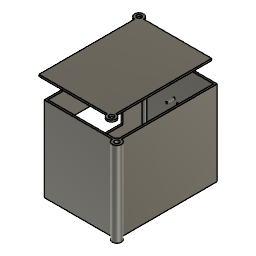
trabajo TEO grupo 5 (Autodesk Fusion 360 design; units mm, degrees)
part number: 2026-06-23-14-01-29-203
Autodesk Fusion 360 part; units mm, degrees
sketch "Boceto1" plane through (0, 0, 0) normal (0, 0, 1) x (1, 0, 0)
  line L0 (0, 0) -> (-75, 0)
  line L1 (-75, 0) -> (-75, -105)
  line L2 (-75, -105) -> (0, -105)
  line L3 (0, -105) -> (0, 0)
  dimension "d1" = 75
  dimension "d2" = 105
  constraint horizontal L0
  constraint vertical L1
  constraint horizontal L2
  constraint vertical L3
  constraint coincident L0.start L3.end
  measures "d1" distance of L0.start L0.end
  measures "d2" distance of L0.start L2.end
extrude "Extruir1" add sketch "Boceto1" along normal blind 90 makes body 1
sketch "Boceto2" plane through (-75, 0, 0) normal (-1, 0, 0) x (0, -1, 0)
  line L0 (0, 0) -> (105, 0)
  line L1 (105, 0) -> (105, 90)
  line L2 (105, 90) -> (0, 90)
  line L3 (0, 90) -> (0, 0)
shell "Vaciado1" thickness 2 outward yes removed faces 1 at (-50, -35, 90) on bodies 1
sketch "Boceto3" plane through (-77, 0, 0) normal (-1, 0, 0) x (0, -1, 0)
  line L0 (-2, -2) -> (107, -2)
  line L1 (107, -2) -> (107, 90)
  line L2 (107, 90) -> (-2, 90)
  line L3 (-2, 90) -> (-2, -2)
sketch "Boceto4" plane through (-75, 0, 0) normal (-1, 0, 0) x (0, -1, 0)
sketch "Boceto5" plane through (0, 0, 0) normal (0, -1, 0) x (1, 0, 0)
  line L0 (-75, 0) -> (0, 0)
  line L1 (0, 0) -> (0, 90)
  line L2 (0, 90) -> (-75, 90)
  line L3 (-75, 90) -> (-75, 0)
  line L4 (-75, 90) -> (0, 90)
  line L5 (-37.5, 90) -> (-37.5, 55)
  line L6 (-37.5, 55) -> (-35, 55)
  line L7 (-37.5, 55) -> (-40, 55)
  line L8 (-40, 55) -> (-40, 40.25)
  line L9 (-40, 55) -> (-35, 55)
  line L10 (-35, 55) -> (-35, 40.25)
  line L11 (-35, 40.25) -> (-40, 40.25)
  line L12 (-40, 40.25) -> (-40, 55)
  dimension "d6" = 35
  dimension "d7" = 2.5
  dimension "d8" = 2.5
  dimension "d9" = 14.75
  constraint coincident L2.end L3.start
  constraint coincident L1.end L2.start
  constraint midpoint L4 L5.start
  constraint perpendicular L2 L5
  constraint perpendicular L5 L6
  constraint perpendicular L5 L7
  constraint perpendicular L7 L8
  constraint horizontal L9
  constraint vertical L10
  constraint horizontal L11
  constraint vertical L12
  measures "d6" distance of L5.start L5.end
  measures "d7" distance of L5.end L6.end
  measures "d8" distance of L5.end L7.end
  measures "d9" distance of L7.end L8.end
extrude "Extruir2" cut sketch "Boceto5" along normal blind 0 and the other way blind 4 contours L6 L7 L8 L9 L10 L11 L12 bodies 1
sketch "Boceto6" plane through (0, 2, 0) normal (0, 1, 0) x (-1, 0, 0)
  line L0 (35, 40.25) -> (35, 55)
  line L1 (35, 55) -> (40, 55)
  line L2 (40, 55) -> (40, 40.25)
  line L3 (40, 40.25) -> (35, 40.25)
  line L4 (-2, -2) -> (77, -2)
  line L5 (77, -2) -> (77, 90)
  line L6 (77, 90) -> (-2, 90)
  line L7 (-2, 90) -> (-2, -2)
  line L8 (37.5, 55) -> (41.7, 55)
  line L9 (37.5, 55) -> (33.3, 55)
  circle A0 centre (32.21, 55) radius 1.09
  circle A1 centre (42.79, 55) radius 1.09
  line L10 (35, 55) -> (35, 51)
  dimension "d14" = 4.2
  dimension "d15" = 4.2
  dimension "d16" = 2.18
  dimension "d17" = 2.18
  dimension "d18" = 4
  constraint midpoint L1 L8.start
  constraint parallel L1 L8
  constraint parallel L1 L9
  constraint coincident L9.end A0
  constraint coincident L8.end A1
  constraint coincident L0.end L1.start
  constraint perpendicular L9 L10
  measures "d14" distance of L8.start L8.end
  measures "d15" distance of L8.start L9.end
  measures "d16" diameter of A0
  measures "d17" diameter of A1
  measures "d18" distance of L0.end L10.end
extrude "Extruir3" add 1 faces at (-36.6667, 0.6667, 55) along direction (0, 0, -1) blind 2.5 on bodies 1 bodies 1
extrude "Extruir4" cut sketch "Boceto6" along normal blind 0 and the other way blind 3 contours A0 bodies 1
extrude "Extruir5" cut sketch "Boceto6" against normal blind 3.5 contours A1 bodies 1
sketch "Boceto7" plane through (0, 0, -2) normal (0, 0, -1) x (1, 0, 0)
  line L0 (2, -2) -> (2, 107)
  line L1 (2, 107) -> (-77, 107)
  line L2 (-77, 107) -> (-77, -2)
  line L3 (-77, -2) -> (2, -2)
sketch "Boceto8" plane through (-75, 0, 0) normal (-1, 0, 0) x (0, -1, 0)
  line L0 (105, 90) -> (0, 90)
  line L1 (52.5, 90) -> (52.5, 60.8734)
  line L2 (52.5, 60.8734) -> (23.5, 60.8734)
  line L3 (52.5, 60.8734) -> (81.5, 60.8734)
  line L4 (23.5, 60.8734) -> (23.5, 25.8734)
  line L5 (23.5, 60.8734) -> (81.5, 60.8734)
  line L6 (81.5, 60.8734) -> (81.5, 25.8734)
  line L7 (81.5, 25.8734) -> (23.5, 25.8734)
  line L8 (23.5, 25.8734) -> (23.5, 60.8734)
  dimension "d27" = 29
  dimension "d28" = 29
  dimension "d29" = 35
  constraint midpoint L0 L1.start
  constraint perpendicular L0 L1
  constraint perpendicular L1 L2
  constraint perpendicular L1 L3
  constraint perpendicular L2 L4
  constraint horizontal L5
  constraint vertical L6
  constraint horizontal L7
  constraint vertical L8
  measures "d27" distance of L1.end L2.end
  measures "d28" distance of L1.end L3.end
  measures "d29" distance of L2.end L4.end
extrude "Extruir6" cut sketch "Boceto8" along normal blind 19 bodies 1
sketch "Boceto9" plane through (0, 0, 0) normal (0, 0, 1) x (-1, 0, 0)
  line L0 (0, 105) -> (0, 0)
  line L1 (0, 0) -> (75, 0)
  line L2 (75, 0) -> (75, 105)
  line L3 (75, 105) -> (0, 105)
  line L4 (37.5, 105) -> (37.5, 0)
  circle A0 centre (37.5, 52.5) radius 9.725
  line L5 (-2, -2, -2) -> (-2, 107, -2)
  line L6 (-2, 107, -2) -> (77, 107, -2)
  line L7 (77, 107, -2) -> (77, -2, -2)
  line L8 (77, -2, -2) -> (-2, -2, -2)
  dimension "d32" = 19.45
  constraint midpoint L3 L4.start
  constraint midpoint L1 L4.end
  constraint midpoint L4 A0.centre
  measures "d32" diameter of A0
extrude "Extruir7" cut sketch "Boceto9" along normal blind -25 and the other way blind 0 contours L4 A0 | L4 A0 bodies 1
sketch "Boceto10" plane through (0, 0, 0) normal (0, 0, 1) x (-1, 0, 0)
  circle A0 centre (37.5, 52.5) radius 9.725
  line L0 (0, 105) -> (0, 0)
  line L1 (0, 0) -> (75, 0)
  line L2 (75, 0) -> (75, 105)
  line L3 (75, 105) -> (0, 105)
  line L4 (30.6188, 59.3721) -> (44.3812, 59.3721)
  line L5 (28.7722, 56.7896) -> (46.2278, 56.7896)
  line L6 (27.775, 52.5) -> (47.225, 52.5)
  line L7 (28.7699, 48.215) -> (46.2301, 48.215)
  line L8 (31.7733, 44.64) -> (43.2267, 44.64)
  constraint coincident A0 L4.start
  constraint coincident A0 L4.end
  constraint horizontal L4
  constraint coincident A0 L5.start
  constraint coincident A0 L5.end
  constraint parallel L4 L5
  constraint coincident A0 L6.start
  constraint coincident A0 L6.end
  constraint parallel L5 L6
  constraint coincident A0 L7.start
  constraint coincident A0 L7.end
  constraint parallel L5 L7
  constraint coincident A0 L8.start
  constraint coincident A0 L8.end
  constraint parallel L7 L8
extrude "Extruir8" add sketch "Boceto10" against normal blind 2 contours A0 L6 L7 | A0 L4 L5 | A0 L8 bodies 1
sketch "Boceto11" plane through (0, 0, 0) normal (0, 0, 1) x (-1, 0, 0)
  arc A0 (43.2267, 44.64) -> (46.2301, 48.215) centre (37.5, 52.5) ccw
  line L0 (43.2267, 44.64) -> (31.7733, 44.64)
  arc A1 (28.7699, 48.215) -> (31.7733, 44.64) centre (37.5, 52.5) ccw
  line L1 (28.7699, 48.215) -> (46.2301, 48.215)
  line L2 (47.225, 52.5) -> (27.775, 52.5)
  arc A2 (28.7722, 56.7896) -> (27.775, 52.5) centre (37.5, 52.5) ccw
  line L3 (28.7722, 56.7896) -> (46.2278, 56.7896)
  arc A3 (47.225, 52.5) -> (46.2278, 56.7896) centre (37.5, 52.5) ccw
  line L4 (44.3812, 59.3721) -> (30.6188, 59.3721)
  arc A4 (44.3812, 59.3721) -> (30.6188, 59.3721) centre (37.5, 52.5) ccw
  line L5 (0, 105) -> (0, 0)
  line L6 (0, 0) -> (75, 0)
  line L7 (75, 0) -> (75, 105)
  line L8 (75, 105) -> (0, 105)
  line L9 (31.0217, 64.79) -> (43.5417, 64.79)
  circle A5 centre (44.9317, 64.79) radius 1.39
  circle A6 centre (29.6317, 64.79) radius 1.39
  line L10 (29.6819, 63.4009) -> (29.6819, 38.6409)
  line L11 (44.9317, 63.4) -> (44.9317, 38.64)
  circle A7 centre (29.6819, 37.2509) radius 1.39
  circle A8 centre (44.9317, 37.25) radius 1.39
  dimension "d39" = 12.52
  dimension "d40" = 2.78
  dimension "d41" = 2.78
  dimension "d42" = 24.76
  dimension "d43" = 24.76
  dimension "d44" = 2.78
  dimension "d45" = 2.78
  constraint horizontal L9
  constraint coincident L9.end A5
  constraint coincident L9.start A6
  constraint coincident A6 L10.start
  constraint perpendicular L1 L10
  constraint coincident A5 L11.start
  constraint vertical L11
  constraint coincident L10.end A7
  constraint coincident L11.end A8
  measures "d39" distance of L9.start L9.end
  measures "d40" diameter of A5
  measures "d41" diameter of A6
  measures "d42" distance of L10.start L10.end
  measures "d43" distance of L11.start L11.end
  measures "d44" diameter of A7
  measures "d45" diameter of A8
extrude "Extruir9" cut sketch "Boceto11" along normal blind -4 and the other way blind 0 contours A5 | A6 | A7 | A8 bodies 1
sketch "Boceto12" plane through (-75, 0, 0) normal (-1, 0, 0) x (0, -1, 0)
  line L0 (23.5, 25.8734) -> (81.5, 25.8734)
  line L1 (52.5, 25.8734) -> (52.5, 23.9434)
  circle A0 centre (52.5, 21.7434) radius 2.2
  dimension "d50" = 1.93
  dimension "d51" = 4.4
  constraint midpoint L0 L1.start
  constraint perpendicular L0 L1
  constraint coincident L1.end A0
  measures "d50" distance of L1.start L1.end
  measures "d51" diameter of A0
extrude "Extruir10" add sketch "Boceto12" against normal blind 19 bodies 1
sketch "Boceto13" plane through (0, 0, 0) normal (0, 0, 1) x (-1, 0, 0)
  line L0 (0, 105) -> (0, 0)
  line L1 (0, 0) -> (75, 0)
  line L2 (75, 0) -> (75, 105)
  line L3 (75, 105) -> (0, 105)
  line L4 (44.3812, 59.3721) -> (30.6188, 59.3721)
  arc A0 (44.3812, 59.3721) -> (30.6188, 59.3721) centre (37.5, 52.5) ccw
  line L5 (47.225, 52.5) -> (27.775, 52.5)
  arc A1 (28.7722, 56.7896) -> (27.775, 52.5) centre (37.5, 52.5) ccw
  line L6 (28.7722, 56.7896) -> (46.2278, 56.7896)
  arc A2 (47.225, 52.5) -> (46.2278, 56.7896) centre (37.5, 52.5) ccw
  arc A3 (43.2267, 44.64) -> (46.2301, 48.215) centre (37.5, 52.5) ccw
  line L7 (43.2267, 44.64) -> (31.7733, 44.64)
  arc A4 (28.7699, 48.215) -> (31.7733, 44.64) centre (37.5, 52.5) ccw
  line L8 (28.7699, 48.215) -> (46.2301, 48.215)
  circle A5 centre (29.6819, 37.2509) radius 1.39
  circle A6 centre (44.9317, 64.79) radius 1.39
  circle A7 centre (44.9317, 37.25) radius 1.39
  circle A8 centre (29.6317, 64.79) radius 1.39
  circle A9 centre (29.6819, 37.2509) radius 1.39
  circle A10 centre (44.9317, 37.25) radius 1.39
  circle A11 centre (44.9317, 64.79) radius 1.39
  circle A12 centre (29.6317, 64.79) radius 1.39
  constraint concentric A5 A9
  constraint concentric A7 A10
  constraint concentric A6 A11
  constraint concentric A8 A12
extrude "Extruir11" add sketch "Boceto13" along normal blind 23 separate body contours A5 A9 | A6 A11 | A7 A10 | A8 A12 makes body 2 at (-46.3199, -37.1808, 15.3333) makes body 3 at (-31.0702, -37.1817, 15.3333) makes body 4 at (-28.2434, -64.8593, 15.3333) makes body 5 at (-46.1524, -65.4548, 7.6667)
extrude "Extruir12" add sketch "Boceto6" along normal blind 0 and the other way blind 10 contours A0 | A1 bodies 1
sketch "Boceto14" plane through (0, 0, -2) normal (0, 0, -1) x (1, 0, 0)
  circle A0 centre (1.9998, 106.9999) radius 5
  circle A1 centre (-76.9997, -1.9997) radius 5
  dimension "d60" = 10
  dimension "d61" = 10
  measures "d60" diameter of A0
  measures "d61" diameter of A1
extrude "Extruir13" add sketch "Boceto14" along normal blind 0 and the other way blind 92 bodies 1
sketch "Boceto15" plane through (0, 0, 90) normal (0, 0, 1) x (-1, 0, 0)
  line L0 (2.5828, 105) -> (75, 105)
  line L1 (75, 105) -> (75, 2.583)
  arc A0 (75, 2.583) -> (72.417, 0) centre (76.9997, -1.9997) ccw
  line L2 (72.417, 0) -> (0, 0)
  line L3 (0, 0) -> (0, 102.4172)
  arc A1 (0, 102.4172) -> (2.5828, 105) centre (-1.9998, 106.9999) ccw
  arc A2 (3.0002, 107) -> (-2, 101.9999) centre (-1.9998, 106.9999) ccw
  line L4 (-2, 101.9999) -> (-2, -2)
  line L5 (-2, -2) -> (71.9997, -2)
  arc A3 (71.9997, -2) -> (77, 3.0003) centre (76.9997, -1.9997) ccw
  line L6 (77, 3.0003) -> (77, 107)
  line L7 (77, 107) -> (3.0002, 107)
  circle A4 centre (76.9997, -1.9997) radius 2.5
  circle A5 centre (-1.9998, 106.9999) radius 2.5
  dimension "d66" = 5
  dimension "d67" = 5
  constraint concentric A0 A4
  constraint concentric A1 A5
  measures "d66" diameter of A4
  measures "d67" diameter of A5
extrude "Extruir14" cut sketch "Boceto15" against normal blind 4 contours A4 | A5 bodies 1
sketch "Boceto16" plane through (0, 0, 90) normal (0, 0, 1) x (-1, 0, 0)
  circle A0 centre (-1.9998, 106.9999) radius 2.5
  circle A1 centre (76.9997, -1.9997) radius 2.5
  line L0 (2.5828, 105) -> (75, 105)
  line L1 (75, 105) -> (75, 2.583)
  arc A2 (75, 2.583) -> (72.417, 0) centre (76.9997, -1.9997) ccw
  line L2 (72.417, 0) -> (0, 0)
  line L3 (0, 0) -> (0, 102.4172)
  arc A3 (0, 102.4172) -> (2.5828, 105) centre (-1.9998, 106.9999) ccw
  arc A4 (3.0002, 107) -> (-2, 101.9999) centre (-1.9998, 106.9999) ccw
  line L4 (-2, 101.9999) -> (-2, -2)
  line L5 (-2, -2) -> (71.9997, -2)
  arc A5 (71.9997, -2) -> (77, 3.0003) centre (76.9997, -1.9997) ccw
  line L6 (77, 3.0003) -> (77, 107)
  line L7 (77, 107) -> (3.0002, 107)
  line L8 (-2, -2) -> (77, -2)
  line L9 (77, -2) -> (77, 107)
  line L10 (77, 107) -> (-2, 107)
  line L11 (-2, 107) -> (-2, -2)
  constraint horizontal L8
  constraint vertical L9
  constraint horizontal L10
  constraint vertical L11
  constraint coincident L6.end L7.start
  constraint coincident L4.end L5.start
extrude "Extruir15" add sketch "Boceto16" along normal blind 2 separate body contours A0 A1 L4 L5 L6 L7 L8 L9 L10 L11 | A0 A4 L10 L11 | A1 A5 L8 L9 | L0 L1 A2 L2 L3 A3 makes body 6
move_body "Desplazar1" bodies 6 to x (1, 0, 0) y (0, 1, 0) z (0, 0, 1) at (-4.0493, -1.7744, 20.8076)
